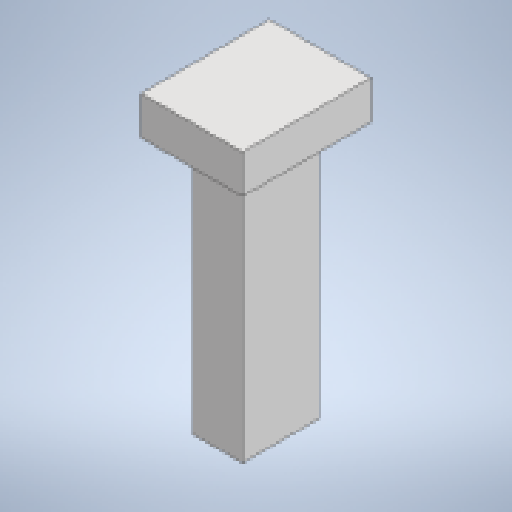
# Autodesk Inventor part: палка
Saved by Autodesk Inventor 2023.1 (Build 271208000, 208)
## iProperties
Created: 2025-01-24
Part Number: палка
Material: Типовые
Document SubType Name: Modeling
Designer: DELL
Density: 1 g/cm^3
Appearance: По умолчанию
Author: DELL
Autodesk Inventor part; units mm, degrees
ref_plane "YZ Plane" through (0, 0, 0) normal (1, 0, 0) x (0, 1, 0)
ref_plane "XZ Plane" through (0, 0, 0) normal (0, 1, 0) x (-1, 0, 0)
ref_plane "XY Plane" through (0, 0, 0) normal (0, 0, 1) x (1, 0, 0)
sketch "Эскиз1" plane through (0, 0, 0) normal (0, 1, 0) x (-1, 0, 0)
  line L0 (2.774, 2.3279) -> (-1.126, 2.3279)
  line L1 (-1.126, 2.3279) -> (-1.126, -3.6721)
  line L2 (-1.126, -3.6721) -> (2.774, -3.6721)
  line L3 (2.774, -3.6721) -> (2.774, 2.3279)
  point P0 (0, 0)
  dimension "d0" = 3.9
  dimension "d1" = 6
  constraints: 8 end point, 2 parallel, 1 horizontal, 1 perpendicular
  measures "d0" distance of L2.end L1.end
  measures "d1" distance of L1.end L0.end
extrude "Выдавливание1" add sketch "Эскиз1" along normal blind 20
sketch "Эскиз2" plane through (0, 20, 0) normal (0, 1, 0) x (1, 0, 0)
  line L0 (1.126, -2.3279) -> (1.126, 3.6721) projected
  line L1 (1.126, 3.6721) -> (-2.774, 3.6721) projected
  line L2 (-2.774, 3.6721) -> (-2.774, -2.3279) projected
  line L3 (-2.774, -2.3279) -> (1.126, -2.3279) projected
  line L4 (3.126, 5.6721) -> (3.126, -4.3279)
  line L5 (3.126, -4.3279) -> (-4.774, -4.3279)
  line L6 (-4.774, -4.3279) -> (-4.774, 5.6721)
  line L7 (-4.774, 5.6721) -> (3.126, 5.6721)
  point P0 (0, 0)
  dimension "d4" = 2
  constraints: 8 end point, 3 other
  measures "d4" distance between parallel lines of L0 L4
extrude "Выдавливание2" add sketch "Эскиз2" along normal blind 3 contours L3 L2 L1 L0 | L4 L5 L6 L7
